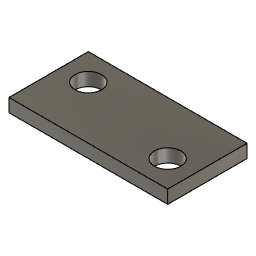
Plate (Autodesk Fusion 360 design; units mm, degrees)
Autodesk Fusion 360 part; units mm, degrees
sketch "Sketch1" plane through (0, 0, 0) normal (0, 0, 1) x (1, 0, 0)
  line L0 (0, 0) -> (60, 0)
  line L1 (60, 0) -> (60, 30)
  line L2 (60, 30) -> (0, 30)
  line L3 (0, 30) -> (0, 0)
  circle A0 centre (10, 20) radius 5
  circle A1 centre (50, 10) radius 5
  dimension "d1" = 60
  dimension "d2" = 30
  dimension "d3" = 10
  dimension "d4" = 10
  dimension "d5" = 10
  dimension "d6" = 10
  dimension "d7" = 10
  dimension "d8" = 10
  constraint horizontal L0
  constraint vertical L1
  constraint horizontal L2
  constraint vertical L3
  constraint coincident L0.start L3.end
  measures "d1" distance of L1.end L2.end
  measures "d2" distance of L0.end L1.end
  measures "d3" diameter of A0
  measures "d4" diameter of A1
  measures "d5" distance of L0 A1.centre
  measures "d6" distance of L1 A1.centre
  measures "d7" distance of L2 A0.centre
  measures "d8" distance of L3 A0.centre
extrude "Extrude1" add sketch "Sketch1" along normal blind 5
named bodies: "Plate"
